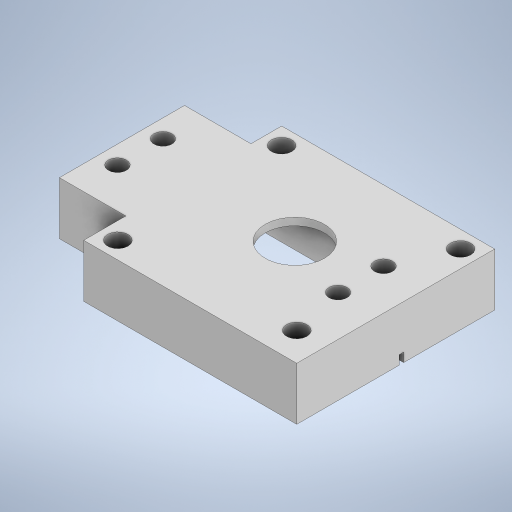
# Autodesk Inventor part: Servo Mount
Saved by Autodesk Inventor 2023 (Build 270158000, 158)
## iProperties
Created: 2023-03-13
Part Number: Servo Mount
Material: Generic
Document SubType Name: Modeling
Designer: tommy
Density: 1 g/cm^3
Appearance: Default
Author: tommy
Autodesk Inventor part; units mm, degrees
ref_plane "YZ Plane" through (0, 0, 0) normal (1, 0, 0) x (0, 1, 0)
ref_plane "XZ Plane" through (0, 0, 0) normal (0, 1, 0) x (-1, 0, 0)
ref_plane "XY Plane" through (0, 0, 0) normal (0, 0, 1) x (1, 0, 0)
sketch "Sketch1" plane through (0, 0, 0) normal (0, 1, 0) x (-1, 0, 0)
  line L0 (0, 0) -> (41.148, 0)
  line L1 (41.148, 0) -> (41.148, -20.32)
  line L2 (41.148, -20.32) -> (0, -20.32)
  line L3 (0, -20.32) -> (0, 0)
  circle A0 centre (45.212, -15.24) radius 2.0193
  circle A1 centre (-4.064, -15.24) radius 2.0193
  circle A2 centre (45.212, -5.08) radius 2.0193
  circle A3 centre (-4.064, -5.08) radius 2.0193
  line L4 (41.148, -9.652) -> (49.276, -9.652)
  line L5 (41.148, -10.668) -> (49.276, -10.668)
  line L6 (-13.1318, -9.652) -> (0, -9.652)
  line L7 (-13.1318, -10.668) -> (0, -10.668)
  line L8 (-13.1318, 3.81) -> (49.276, 3.81)
  line L9 (49.276, 3.81) -> (49.276, -24.13)
  line L10 (49.276, -24.13) -> (-13.1318, -24.13)
  line L11 (-13.1318, -30.9945) -> (-13.1318, 13.2145)
  line L12 (-6.155, -5.4575) -> (-6.0508, -5.4409)
  line L13 (-6.155, -5.4575) -> (-6.0508, -5.4409)
  line L14 (20.574, -20.32) -> (20.574, 0)
  circle A4 centre (10.668, -10.16) radius 6.604
  circle A5 centre (-6.7818, 6.8645) radius 2.0193
  circle A6 centre (30.6451, 9.4045) radius 2.0193
  circle A7 centre (30.6451, -27.1845) radius 2.0193
  line L15 (10.668, -30.9945) -> (34.4551, -30.9945)
  line L16 (-8.128, -30.9945) -> (34.4551, -30.9945)
  circle A8 centre (-9.3218, -27.1845) radius 2.0193
  line L17 (34.4424, -30.9945) -> (-13.1318, -30.9945)
  line L18 (34.4424, -24.13) -> (34.4424, -30.9945)
  line L19 (34.4424, 13.2145) -> (34.4424, 3.81)
  circle A9 centre (30.6451, 9.4045) radius 2.286
  circle A10 centre (-6.7818, 6.8645) radius 2.286
  circle A11 centre (-9.3218, -27.1845) radius 2.286
  circle A12 centre (30.6451, -27.1845) radius 2.286
  line L20 (34.4424, 3.81) -> (-13.1318, 3.81)
  line L21 (34.4424, 13.2145) -> (-13.1318, 13.2145)
  point P0 (20.574, -10.16)
  point P1 (34.4424, -30.9945)
  point P2 (-11.5492, -24.13)
  point P3 (-7.0944, -24.13)
  dimension "d0" = 41.148
  dimension "d1" = 20.32
  dimension "d4" = 4.0386
  dimension "d5" = 4.0386
  dimension "d18" = 4.064
  dimension "d19" = 4.064
  dimension "d52" = 8.128
  dimension "d53" = 13.1318
  dimension "d54" = 3.81
  dimension "d55" = 3.81
  dimension "d59" = 9.906
  dimension "d60" = 13.208
  dimension "d79" = 4.0386
  dimension "d80" = 4.0386
  dimension "d81" = 4.0386
  dimension "d82" = 4.0386
  dimension "d84" = 3.81
  dimension "d91" = 4.572
  dimension "d92" = 4.572
  dimension "d93" = 4.572
  dimension "d94" = 4.572
  dimension "d96" = 3.81
  dimension "d97" = 3.81
  dimension "d98" = 6.35
  dimension "d100" = 6.35
  dimension "d101" = 9.4045
  dimension "d102" = 47.5742
  dimension "d103" = 47.5742
  constraints: 44 end point, 13 point on line, 12 centre point, 5 coincident, 4 horizontal, 4 parallel, 4 perpendicular, 3 midpoint, 3 other
  measures "d0" distance of L1.end L2.end
  measures "d1" distance of L0.end L1.end
  measures "d4" diameter of A0
  measures "d5" diameter of A1
  measures "d18" distance from line of L1 A0.centre
  measures "d19" distance from line of L3 A1.centre
  measures "d52" distance between parallel lines of L1 L9
  measures "d53" distance between parallel lines of L11 L3
  measures "d54" distance between parallel lines of L2 L10
  measures "d55" distance between parallel lines of L8 L0
  measures "d59" distance of point (20.574, -10.16) point (10.668, -10.16)
  measures "d60" diameter of A4
  measures "d79" diameter of A6
  measures "d80" diameter of A7
  measures "d81" diameter of A8
  measures "d82" diameter of A5
  measures "d84" distance from line of L15 A7.centre
  measures "d91" diameter of A9
  measures "d92" diameter of A10
  measures "d93" diameter of A11
  measures "d94" diameter of A12
  measures "d96" distance from line of L17 A8.centre
  measures "d97" distance from line of L11 A8.centre
  measures "d98" distance from line of L11 A5.centre
  measures "d100" distance from line of L21 A5.centre
  measures "d101" distance between parallel lines of L8 L21
  measures "d102" distance between parallel lines of L19 L11
  measures "d103" distance between parallel lines of L11 L18
extrude "Extrusion10" add sketch "Sketch1" along normal blind 11.811 contours L3 L6 L11 L8 L9 L4 L1 L0 | L0 L14 L2 L3 | L0 L1 L2 L14 | L3 L7 L11 L6 | L2 L1 L5 L9 L10 L11 L7 L3 | L4 L9 L5 L1 | L11 L21 L19 L8 | L10 L18 L15 L16 L17 L11
extrude "Extrusion11" cut sketch "Sketch1" along normal blind 10.16 contours L0 L14 L2 L3 | L0 L1 L2 L14
extrude "Extrusion12" cut sketch "Sketch1" along normal blind 2.032 contours L3 L7 L11 L6 | L4 L9 L5 L1
body "Solid4"
